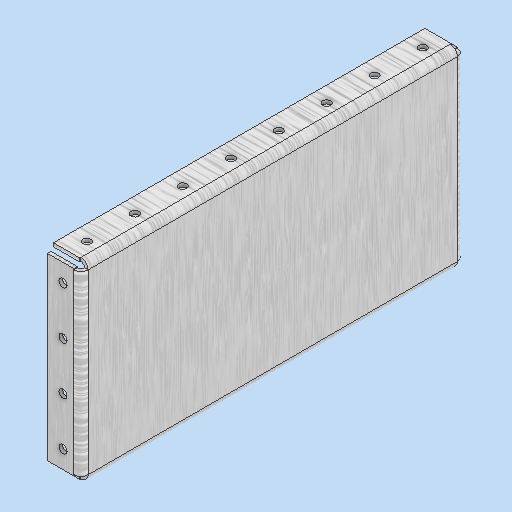
# Autodesk Inventor part: backshort_0.1
Saved by Autodesk Inventor 2026.2 (Build 302298000, 298)
## iProperties
Created: 2026-03-02
Part Number: backshort_0.1
Material: Aluminum 5052
Document SubType Name: Sheet Metal
Designer: alpgo
Density: 2.68 g/cm^3
Sheet Metal Rule: Default_mm
Appearance: Satin - Brushed Heavy
Flat Pattern Width: 10.2786 cm
Flat Pattern Length: 18.2786 cm
Flat Pattern Area: 187.878 cm^2
Sheet Metal Width: 102,786 mm
Sheet Metal Length: 182,786 mm
Sheet Metal Area: 18787,796 mm^2
Author: alpgo
Autodesk Inventor part; units mm, degrees
note: some values were not read from the file. Chosen so that the rebuilt part matches the saved one: corner form of "Plate2".
ref_plane "YZ Plane" through (0, 0, 0) normal (1, 0, 0) x (0, 1, 0)
ref_plane "XZ Plane" through (0, 0, 0) normal (0, 1, 0) x (-1, 0, 0)
ref_plane "XY Plane" through (0, 0, 0) normal (0, 0, 1) x (1, 0, 0)
sketch "Sketch1" plane through (0, 0, 0) normal (1, 0, 0) x (0, 1, 0)
  line L0 (-40, 80) -> (40, 80)
  line L1 (40, 80) -> (40, -80)
  line L2 (40, -80) -> (-40, -80)
  line L3 (-40, -80) -> (-40, 80)
  line L4 (-40, 80) -> (40, -80) construction
  line L5 (40, 80) -> (-40, -80) construction
  point P0 (0, 0)
  dimension "d0" = 160
  dimension "d1" = 80
  measures "d0" distance of L0.end L1.end
  measures "d1" distance of L1.end L2.end
extrude "Plate1" add sketch "Sketch1" along normal mid plane 1.5
sketch "Sketch2" plane through (0.75, 38.5, -80) normal (0, 1, 0) x (-1, 0, 0)
  line L0 (0, 160) -> (0, 0)
  line L1 (0, 0) -> (14, 0)
  line L2 (14, 0) -> (14, 160)
  line L3 (14, 160) -> (0, 160)
  constraints: 6 end point, 1 horizontal, 1 perpendicular, 1 vertical
edge flange "Flange1" height 14 angle 90 thickness 1.5 bend radius 1.5 thickness toward (0, 1, 0) relief tear relief width 1.5 relief depth 0.75 corner gap 1.5 corner form 2 edges at (-0.75, 40, 0) (-0.75, 0, 80) (-0.75, -40, 0) (-0.75, 0, -80) wall of the first edge with corners at (0.75, 38.5, 80) (0.75, 38.5, -80) (-13.25, 38.5, -80) (-13.25, 38.5, 80)
bend "Bend1"
corner "Corner1"
sketch "Sketch3" plane through (-13.25, -40, 77.4393) normal (0, -1, 0) x (1, 0, 0)
  circle A0 centre (6.5, -7.4393) radius 1.7
  line L0 (0, 0) -> (11, 0) projected
  line L1 (0, -154.8787) -> (0, 0) projected
  line L2 (11, 2.5607) -> (0, 2.5607) projected
  line L3 (11, 1.0607) -> (0, 1.0607) projected
  point P0 (13.25, -77.4393)
  point P1 (5.5, 0)
  point P2 (5.5, 2.5607)
  dimension "d13" = 3.4
  dimension "d15" = 6.5
  dimension "d32" = 8.5
  constraints: 2 midpoint, 1 centre point
  measures "d13" diameter of A0
  measures "d15" distance from line of L1 A0.centre
  measures "d32" distance from line of A0.centre L3
extrude "Cut1" cut sketch "Sketch3" against normal blind 1.5
pattern_linear "Rectangular Pattern1" count 8 spacing 20 along (0, 0, -1) of "Cut1"
mirror "Mirror1" about plane through (0, 0, 0) normal (0, 1, 0) of "Cut1", "Rectangular Pattern1"
sketch "Sketch4" plane through (-13.25, 37.4393, 80) normal (0, 0, 1) x (1, 0, 0)
  circle A0 centre (6.5, -67.4393) radius 1.7
  line L0 (11, -74.8787) -> (0, -74.8787) projected
  line L1 (0, -74.8787) -> (0, 0) projected
  line L2 (0, -77.4393) -> (11, -77.4393) projected
  point P0 (13.25, -37.4393)
  dimension "d21" = 3.4
  dimension "d23" = 6.5
  dimension "d33" = 10
  constraints: 1 centre point
  measures "d21" diameter of A0
  measures "d23" distance from line of L1 A0.centre
  measures "d33" distance from line of L2 A0.centre
extrude "Cut2" cut sketch "Sketch4" against normal through all
pattern_linear "Rectangular Pattern2" count 4 spacing 20 along (0, 1, 0) of "Cut2"
equation "\"d16\" = Thickness"
equation "\"d24\" = Thickness"
equation "\"d2\" = Thickness"
equation "\"d3\" = BendReliefWidth"
equation "\"d4\" = BendReliefDepth"
equation "\"d5\" = MinimumRemnant"
equation "\"d6\" = TransitionRadius"
equation "\"d9\" = BendRadius"
equation "\"d10\" = CornerReliefSize"
equation "\"d11\" = GapSize"
equation "\"d12\" = JacobiRadiusSize"
equation "\"BendRadius\" = Thickness"
equation "\"BendReliefWidth\" = Thickness"
equation "\"BendReliefDepth\" = 0.5 * Thickness"
equation "\"CornerReliefSize\" = 4 * Thickness"
equation "\"MinimumRemnant\" = 2 * Thickness"
equation "\"TransitionRadius\" = BendRadius"
equation "\"JacobiRadiusSize\" = BendRadius"
equation "\"GapSize\" = Thickness"
equation "\"Thickness\" = 1.5"
body "Solid1"
